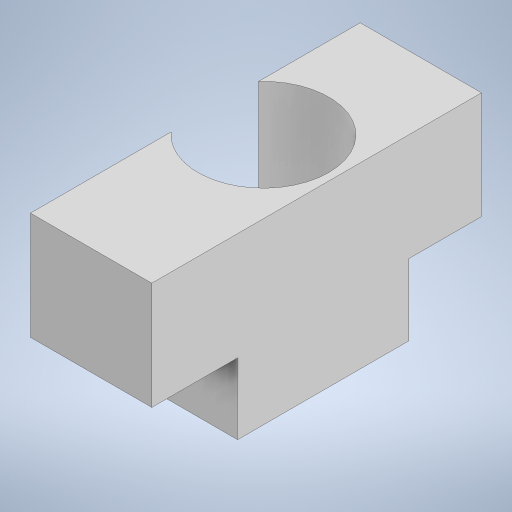
# Autodesk Inventor part: rotary encoder mount
Saved by Autodesk Inventor 2024.2 (Build 282272000, 272)
## iProperties
Created: 2024-09-09
Part Number: rotary encoder mount
Material: Generic
Document SubType Name: Modeling
Designer: Tom
Density: 1 g/cm^3
Appearance: Default
Author: Tom
Autodesk Inventor part; units mm, degrees
ref_plane "YZ Plane" through (0, 0, 0) normal (1, 0, 0) x (0, 1, 0)
ref_plane "XZ Plane" through (0, 0, 0) normal (0, 1, 0) x (-1, 0, 0)
ref_plane "XY Plane" through (0, 0, 0) normal (0, 0, 1) x (1, 0, 0)
sketch "Sketch1" plane through (0, 0, 0) normal (0, 1, 0) x (-1, 0, 0)
  line L0 (0, 0) -> (101.6, 0)
  line L1 (101.6, 0) -> (101.6, -101.6)
  line L2 (101.6, -101.6) -> (0, -101.6)
  line L3 (0, -101.6) -> (0, 0)
  circle A0 centre (50.8, -50.8) radius 5.461
  dimension "d0" = 101.6
  dimension "d1" = 101.6
  dimension "d2" = 10.922
  constraints: 8 end point, 2 parallel, 1 centre point, 1 horizontal, 1 perpendicular
  measures "d0" distance of L0.start L0.end
  measures "d1" distance of L2.end L0.start
  measures "d2" diameter of A0
extrude "Extrusion1" add sketch "Sketch1" along normal blind 4.7625
sketch "Sketch2" plane through (0, 4.7625, 0) normal (0, 1, 0) x (1, 0, 0)
  line L0 (-101.6, 0) -> (0, 0) projected
  line L1 (-76.2, 0) -> (0, 0)
  line L2 (0, 0) -> (0, 33.5923)
  line L3 (0, 33.5923) -> (-76.2, 33.5923)
  line L4 (-76.2, 33.5923) -> (-76.2, 0)
  line L5 (-101.6, 101.6) -> (-101.6, 0) projected
  line L6 (0, 0) -> (0, 101.6) projected
  line L7 (0, 101.6) -> (-101.6, 101.6) projected
  line L8 (-101.6, 76.2) -> (0, 76.2)
  line L9 (0, 76.2) -> (0, 101.6)
  line L10 (0, 101.6) -> (-101.6, 101.6)
  line L11 (-101.6, 101.6) -> (-101.6, 76.2)
  circle A0 centre (-50.8, 50.8) radius 5.461 projected
  line L12 (0, 76.2) -> (-38.1, 76.2)
  line L13 (-38.1, 76.2) -> (-38.1, 33.5923)
  line L14 (-38.1, 33.5923) -> (0, 33.5923)
  line L15 (0, 33.5923) -> (0, 76.2)
  point P0 (0, 76.2)
  dimension "d5" = 25.4
  dimension "d6" = 0
  dimension "d9" = 25.4
  constraints: 24 end point, 6 parallel, 3 horizontal, 3 perpendicular, 2 point on line, 1 midpoint
  measures "d5" distance between parallel lines of L5 L4
  measures "d6" distance between parallel lines of L6 L2
  measures "d9" distance from line of A0.centre L8
extrude "Extrusion2" cut sketch "Sketch2" against normal through all contours L4 L3 L2 L0 | L5 L7 L6 L8 | L8 L6 L3 L13
sketch "Sketch3" plane through (0, 4.7625, 0) normal (0, 1, 0) x (1, 0, 0)
  line L0 (-93.6015, 4.7625) -> (-89.5375, 4.7625)
  line L1 (-89.5375, 4.7625) -> (-89.5375, 71.4375)
  line L2 (-89.5375, 71.4375) -> (-93.6015, 71.4375)
  line L3 (-93.6015, 71.4375) -> (-93.6015, 4.7625)
  line L4 (-101.6, 0) -> (-76.2, 0) projected
  line L5 (-101.6, 76.2) -> (-101.6, 0) projected
  line L6 (-38.1, 76.2) -> (-101.6, 76.2) projected
  line L7 (-83.6041, 71.4375) -> (-83.6041, 4.7625)
  line L8 (-79.5401, 71.4375) -> (-83.6041, 71.4375)
  line L9 (-79.5401, 4.7625) -> (-79.5401, 71.4375)
  line L10 (-83.6041, 4.7625) -> (-79.5401, 4.7625)
  line L11 (-73.6067, 71.4375) -> (-73.6067, 4.7625)
  line L12 (-69.5427, 71.4375) -> (-73.6067, 71.4375)
  line L13 (-69.5427, 4.7625) -> (-69.5427, 71.4375)
  line L14 (-73.6067, 4.7625) -> (-69.5427, 4.7625)
  line L15 (-63.6092, 71.4375) -> (-63.6092, 4.7625)
  line L16 (-59.5452, 71.4375) -> (-63.6092, 71.4375)
  line L17 (-59.5452, 4.7625) -> (-59.5452, 71.4375)
  line L18 (-63.6092, 4.7625) -> (-59.5452, 4.7625)
  point P0 (0, 0)
  dimension "d10" = 4.064
  dimension "d11" = 4.7625
  dimension "d12" = 7.9985
  dimension "d14" = 4.7625
  dimension "d17" = 9.9974
  constraints: 32 end point, 2 horizontal, 2 parallel, 1 perpendicular, 24 other
  measures "d10" distance between parallel lines of L1 L3
  measures "d11" distance between parallel lines of L4 L0
  measures "d12" distance between parallel lines of L5 L3
  measures "d14" distance between parallel lines of L6 L2
  measures "d17" distance of L2.end L7.start
extrude "Extrusion3" cut sketch "Sketch3" against normal through all
sketch "Sketch4" plane through (0, 4.7625, 0) normal (0, 1, 0) x (1, 0, 0)
  circle A0 centre (-50.8, 42.9006) radius 0.9525
  circle A1 centre (-50.8, 50.8) radius 5.461 projected
  point P0 (0, 0)
  dimension "d24" = 1.905
  dimension "d25" = 0
  dimension "d26" = 7.8994
  constraints: 1 centre point
  measures "d24" diameter of A0
  measures "d25" horizontal distance of A1.centre A0.centre
  measures "d26" distance of A1.centre A0.centre
extrude "Extrusion4" cut sketch "Sketch4" against normal through all contours A0
sketch "Sketch5" plane through (0, 4.7625, 0) normal (0, 1, 0) x (1, 0, 0)
  line L0 (-101.6, 0) -> (-76.2, 0) projected
  line L1 (-38.1, 76.2) -> (-101.6, 76.2) projected
  line L2 (-101.6, 0) -> (-59.2938, 0)
  line L3 (-59.2938, 0) -> (-59.2938, 76.2)
  line L4 (-59.2938, 76.2) -> (-101.6, 76.2)
  line L5 (-101.6, 76.2) -> (-101.6, 0)
  point P0 (0, 0)
  constraints: 8 end point, 2 parallel, 1 horizontal, 1 perpendicular, 1 point on line
extrude "Extrusion5" cut sketch "Sketch5" against normal through all
sketch "Sketch6" plane through (0, 4.7625, 0) normal (0, 1, 0) x (1, 0, 0)
  circle A0 centre (-50.8, 50.8) radius 5.461 projected
  line L0 (-59.2938, 76.2) -> (-59.2938, 33.5923) projected
  line L1 (-59.2938, 33.5923) -> (-38.1, 33.5923) projected
  line L2 (-38.1, 33.5923) -> (-38.1, 76.2) projected
  line L3 (-38.1, 76.2) -> (-59.2938, 76.2) projected
  circle A1 centre (-50.8, 42.9006) radius 0.9525 projected
  point P0 (0, 0)
extrude "Extrusion6" add sketch "Sketch6" along normal blind 15.24
sketch "Sketch7" plane through (0, 20.0025, 0) normal (0, 1, 0) x (1, 0, 0)
  circle A0 centre (-50.8, 50.8) radius 5.461 projected
  circle A1 centre (-50.8, 50.8) radius 11.43
  point P0 (0, 0)
  dimension "d33" = 22.86
  constraints: 1 centre point, 1 coincident
  measures "d33" diameter of A1
extrude "Extrusion7" cut sketch "Sketch7" against normal blind 14.986
sketch "Sketch10" plane through (0, 0, 0) normal (0, -1, 0) x (1, 0, 0)
  line L0 (-59.2938, -76.2) -> (-38.1, -76.2) projected
  line L1 (-38.1, -76.2) -> (-38.1, -33.5923) projected
  line L2 (-59.2938, -76.2) -> (-38.1, -76.2)
  line L3 (-38.1, -76.2) -> (-38.1, -63.5)
  line L4 (-38.1, -63.5) -> (-59.2938, -63.5)
  line L5 (-59.2938, -63.5) -> (-59.2938, -76.2)
  point P0 (0, 0)
  dimension "d36" = 12.7
  constraints: 8 end point, 2 parallel, 1 horizontal, 1 perpendicular, 1 point on line
  measures "d36" distance between parallel lines of L0 L4
extrude "Extrusion8" cut sketch "Sketch10" against normal blind 14.986
sketch "Sketch11" plane through (-59.2938, 0, -33.5923) normal (0, 0, 1) x (1, 0, 0)
  line L0 (21.1938, 20.0025) -> (0, 20.0025) projected
  line L1 (21.1938, 20.0025) -> (21.1938, 14.986) projected
  line L2 (0, 20.0025) -> (21.1938, 20.0025)
  line L3 (21.1938, 20.0025) -> (21.1938, 14.9225)
  line L4 (21.1938, 14.9225) -> (0, 14.9225)
  line L5 (0, 14.9225) -> (0, 20.0025)
  point P0 (59.2938, 0)
  point P1 (21.1938, 14.986)
  dimension "d39" = 5.08
  constraints: 8 end point, 2 parallel, 1 horizontal, 1 perpendicular, 1 point on line
  measures "d39" distance between parallel lines of L0 L4
extrude "Extrusion9" add sketch "Sketch11" along normal blind 14.986
sketch "Sketch12" plane through (0, 0, 0) normal (0, -1, 0) x (1, 0, 0)
  line L0 (-59.2938, -63.5) -> (-38.1, -63.5) projected
  line L1 (-38.1, -63.5) -> (-38.1, -33.5923) projected
  line L2 (-38.1, -33.5923) -> (-59.2938, -33.5923) projected
  line L3 (-59.2938, -33.5923) -> (-59.2938, -63.5) projected
  circle A0 centre (-50.8, -42.9006) radius 0.9525 projected
  circle A1 centre (-50.8, -50.8) radius 5.461 projected
  point P0 (0, 0)
extrude "Extrusion10" cut sketch "Sketch12" against normal blind 2.54
sketch "Sketch13" plane through (0, 20.0025, 0) normal (0, 1, 0) x (1, 0, 0)
  arc A0 (-59.2938, 43.1515) -> (-59.2938, 58.4485) centre (-50.8, 50.8) ccw projected
  line L0 (-59.2938, 43.1515) -> (-59.2938, 18.6063) projected
  line L1 (-38.1, 18.6063) -> (-59.2938, 18.6063) projected
  line L2 (-38.1, 76.2) -> (-38.1, 18.6063) projected
  line L3 (-38.1, 76.2) -> (-59.2938, 76.2) projected
  line L4 (-59.2938, 76.2) -> (-59.2938, 58.4485) projected
  point P0 (0, 0)
extrude "Extrusion11" add sketch "Sketch13" along normal blind 13.716
body "Solid1"
